Autodesk Fusion 360 part; units mm, degrees
(part 2 of 2)
  spline S17 degree 5 poles (28.5555, 1.0566) (28.5421, 1.0647) (28.5154, 1.0808) (28.4753, 1.1049) (28.4218, 1.1368) (28.3548, 1.1763) (28.2877, 1.2154) (28.2205, 1.2541) (28.1532, 1.2924) (28.0858, 1.3303) (28.0183, 1.3678) (27.9507, 1.4049) (27.883, 1.4416) (27.8153, 1.4778) (27.7474, 1.5136) (27.6795, 1.549) (27.6114, 1.584) (27.5433, 1.6186) (27.4751, 1.6527) (27.4068, 1.6864) (27.3384, 1.7197) (27.27, 1.7525) (27.2015, 1.7849) (27.1329, 1.8169) (27.0642, 1.8484) (26.9954, 1.8794) (26.9266, 1.91) (26.8577, 1.9401) (26.7887, 1.9698) (26.7197, 1.999) (26.6506, 2.0277) (26.5814, 2.056) (26.5122, 2.0837) (26.4429, 2.111) (26.3735, 2.1378) (26.3041, 2.1641) (26.2347, 2.1899) (26.1651, 2.2152) (26.0955, 2.24) (26.0259, 2.2643) (25.9562, 2.288) (25.8865, 2.3112) (25.8167, 2.3339) (25.7469, 2.356) (25.677, 2.3776) (25.6071, 2.3986) (25.5372, 2.4191) (25.4672, 2.4389) (25.3972, 2.4583) (25.3272, 2.477) (25.2571, 2.4951) (25.187, 2.5126) (25.1169, 2.5294) (25.0467, 2.5455) (24.9766, 2.5609) (24.9064, 2.5757) (24.8362, 2.5899) (24.766, 2.6035) (24.6958, 2.6165) (24.6256, 2.6287) (24.5554, 2.6401) (24.4852, 2.6504) (24.415, 2.6597) (24.3448, 2.6678) (24.2747, 2.6751) (24.2046, 2.6816) (24.1345, 2.6875) (24.0645, 2.693) (23.9945, 2.6977) (23.9245, 2.701) (23.8548, 2.7021) (23.7991, 2.7005) (23.7574, 2.6976) (23.7296, 2.6948) (23.7158, 2.6932) knots -1 -1 -1 -1 -1 -1 -0.98571429 -0.97142857 -0.95714286 -0.94285714 -0.92857143 -0.91428571 -0.9 -0.88571429 -0.87142857 -0.85714286 -0.84285714 -0.82857143 -0.81428571 -0.8 -0.78571429 -0.77142857 -0.75714286 -0.74285714 -0.72857143 -0.71428571 -0.7 -0.68571429 -0.67142857 -0.65714286 -0.64285714 -0.62857143 -0.61428571 -0.6 -0.58571429 -0.57142857 -0.55714286 -0.54285714 -0.52857143 -0.51428571 -0.5 -0.48571429 -0.47142857 -0.45714286 -0.44285714 -0.42857143 -0.41428571 -0.4 -0.38571429 -0.37142857 -0.35714286 -0.34285714 -0.32857143 -0.31428571 -0.3 -0.28571429 -0.27142857 -0.25714286 -0.24285714 -0.22857143 -0.21428571 -0.2 -0.18571429 -0.17142857 -0.15714286 -0.14285714 -0.12857143 -0.11428571 -0.1 -0.08571429 -0.07142857 -0.05714286 -0.04285714 -0.02857143 -0.01428571 0 0 0 0 0 0
  line L17 (23.7158, 2.6932) -> (22.924, 2.6037)
  arc A35 (21.1843, 3.8942) -> (22.924, 2.6037) centre (22.7456, 4.1812) ccw
  arc A36 (21.1843, 3.8942) -> (21.0619, 4.5091) centre (0, 0) ccw
  arc A37 (22.1754, 6.3671) -> (21.0619, 4.5091) centre (22.6143, 4.8415) ccw
  line L18 (22.1754, 6.3671) -> (22.9412, 6.5874)
  spline S18 degree 5 poles (22.9412, 6.5874) (22.9546, 6.5912) (22.9813, 6.5993) (23.0209, 6.6126) (23.073, 6.6324) (23.137, 6.6601) (23.2003, 6.69) (23.2632, 6.7211) (23.3258, 6.7529) (23.3883, 6.7853) (23.4506, 6.8181) (23.5126, 6.8516) (23.5743, 6.886) (23.6356, 6.9214) (23.6965, 6.9578) (23.757, 6.9952) (23.8172, 7.0334) (23.8771, 7.0722) (23.9368, 7.1116) (23.9962, 7.1516) (24.0554, 7.1921) (24.1143, 7.2332) (24.1729, 7.2749) (24.2313, 7.3173) (24.2893, 7.3603) (24.3472, 7.4038) (24.4047, 7.4479) (24.462, 7.4926) (24.519, 7.5377) (24.5758, 7.5834) (24.6323, 7.6296) (24.6886, 7.6762) (24.7447, 7.7234) (24.8005, 7.771) (24.856, 7.8192) (24.9113, 7.8678) (24.9663, 7.9168) (25.0211, 7.9664) (25.0757, 8.0163) (25.13, 8.0668) (25.1841, 8.1176) (25.2379, 8.1689) (25.2915, 8.2206) (25.3448, 8.2728) (25.3979, 8.3254) (25.4508, 8.3784) (25.5034, 8.4318) (25.5557, 8.4856) (25.6079, 8.5398) (25.6597, 8.5944) (25.7114, 8.6493) (25.7628, 8.7047) (25.8139, 8.7605) (25.8649, 8.8166) (25.9155, 8.8732) (25.966, 8.9301) (26.0162, 8.9873) (26.0661, 9.045) (26.1158, 9.103) (26.1653, 9.1613) (26.2145, 9.2201) (26.2635, 9.2791) (26.3122, 9.3386) (26.3607, 9.3983) (26.409, 9.4584) (26.457, 9.5189) (26.5047, 9.5797) (26.5523, 9.6408) (26.5995, 9.7023) (26.6466, 9.7641) (26.6933, 9.8262) (26.7306, 9.8762) (26.7584, 9.9138) (26.7769, 9.939) (26.7861, 9.9516) knots 0 0 0 0 0 0 0.01428571 0.02857143 0.04285714 0.05714286 0.07142857 0.08571429 0.1 0.11428571 0.12857143 0.14285714 0.15714286 0.17142857 0.18571429 0.2 0.21428571 0.22857143 0.24285714 0.25714286 0.27142857 0.28571429 0.3 0.31428571 0.32857143 0.34285714 0.35714286 0.37142857 0.38571429 0.4 0.41428571 0.42857143 0.44285714 0.45714286 0.47142857 0.48571429 0.5 0.51428571 0.52857143 0.54285714 0.55714286 0.57142857 0.58571429 0.6 0.61428571 0.62857143 0.64285714 0.65714286 0.67142857 0.68571429 0.7 0.71428571 0.72857143 0.74285714 0.75714286 0.77142857 0.78571429 0.8 0.81428571 0.82857143 0.84285714 0.85714286 0.87142857 0.88571429 0.9 0.91428571 0.92857143 0.94285714 0.95714286 0.97142857 0.98571429 1 1 1 1 1 1
  arc A38 (26.7861, 9.9516) -> (25.9775, 11.9038) centre (0, 0) ccw
  spline S19 degree 5 poles (25.9775, 11.9038) (25.962, 11.9062) (25.9312, 11.9109) (25.8849, 11.9178) (25.8232, 11.9268) (25.7462, 11.9377) (25.6693, 11.9481) (25.5924, 11.9582) (25.5156, 11.9678) (25.4388, 11.977) (25.3621, 11.9858) (25.2855, 11.9942) (25.2089, 12.0022) (25.1324, 12.0098) (25.056, 12.0169) (24.9797, 12.0236) (24.9034, 12.0299) (24.8273, 12.0358) (24.7512, 12.0412) (24.6752, 12.0462) (24.5993, 12.0508) (24.5235, 12.0549) (24.4478, 12.0586) (24.3722, 12.0619) (24.2967, 12.0647) (24.2213, 12.0671) (24.146, 12.069) (24.0708, 12.0704) (23.9958, 12.0715) (23.9208, 12.072) (23.846, 12.0721) (23.7712, 12.0717) (23.6967, 12.0709) (23.6222, 12.0696) (23.5479, 12.0678) (23.4737, 12.0655) (23.3996, 12.0628) (23.3257, 12.0595) (23.2519, 12.0558) (23.1783, 12.0516) (23.1048, 12.0469) (23.0315, 12.0416) (22.9584, 12.0359) (22.8854, 12.0296) (22.8126, 12.0228) (22.74, 12.0154) (22.6676, 12.0076) (22.5953, 11.9992) (22.5232, 11.9902) (22.4513, 11.9808) (22.3796, 11.9707) (22.3082, 11.96) (22.237, 11.9487) (22.166, 11.9367) (22.0953, 11.9241) (22.0248, 11.9109) (21.9545, 11.8972) (21.8845, 11.8829) (21.8146, 11.868) (21.7451, 11.8524) (21.6759, 11.836) (21.6071, 11.8187) (21.5387, 11.8004) (21.4708, 11.7811) (21.4032, 11.761) (21.3359, 11.7401) (21.2689, 11.7188) (21.2021, 11.697) (21.1356, 11.6746) (21.0698, 11.6509) (21.0049, 11.6252) (20.954, 11.6024) (20.9166, 11.5838) (20.8921, 11.5706) (20.8798, 11.5639) knots -1 -1 -1 -1 -1 -1 -0.98571429 -0.97142857 -0.95714286 -0.94285714 -0.92857143 -0.91428571 -0.9 -0.88571429 -0.87142857 -0.85714286 -0.84285714 -0.82857143 -0.81428571 -0.8 -0.78571429 -0.77142857 -0.75714286 -0.74285714 -0.72857143 -0.71428571 -0.7 -0.68571429 -0.67142857 -0.65714286 -0.64285714 -0.62857143 -0.61428571 -0.6 -0.58571429 -0.57142857 -0.55714286 -0.54285714 -0.52857143 -0.51428571 -0.5 -0.48571429 -0.47142857 -0.45714286 -0.44285714 -0.42857143 -0.41428571 -0.4 -0.38571429 -0.37142857 -0.35714286 -0.34285714 -0.32857143 -0.31428571 -0.3 -0.28571429 -0.27142857 -0.25714286 -0.24285714 -0.22857143 -0.21428571 -0.2 -0.18571429 -0.17142857 -0.15714286 -0.14285714 -0.12857143 -0.11428571 -0.1 -0.08571429 -0.07142857 -0.05714286 -0.04285714 -0.02857143 -0.01428571 0 0 0 0 0 0
  line L19 (20.8798, 11.5639) -> (20.1826, 11.1781)
  arc A39 (18.0815, 11.7046) -> (20.1826, 11.1781) centre (19.4141, 12.5673) ccw
  arc A40 (18.0815, 11.7046) -> (17.7331, 12.226) centre (0, 0) ccw
  arc A41 (18.0508, 14.3686) -> (17.7331, 12.226) centre (19.0401, 13.127) ccw
  line L20 (18.0508, 14.3686) -> (18.674, 14.8652)
  spline S20 degree 5 poles (18.674, 14.8652) (18.6849, 14.8739) (18.7065, 14.8915) (18.738, 14.919) (18.7785, 14.9572) (18.8271, 15.0073) (18.8742, 15.0591) (18.9204, 15.1119) (18.966, 15.1653) (19.0114, 15.2191) (19.0564, 15.2733) (19.1008, 15.3279) (19.1447, 15.3833) (19.1877, 15.4395) (19.2301, 15.4965) (19.2717, 15.5541) (19.3127, 15.6124) (19.3532, 15.6712) (19.3932, 15.7305) (19.4328, 15.7902) (19.472, 15.8502) (19.5106, 15.9108) (19.5489, 15.9717) (19.5866, 16.0332) (19.6238, 16.0951) (19.6605, 16.1575) (19.6968, 16.2203) (19.7326, 16.2834) (19.768, 16.347) (19.803, 16.4109) (19.8376, 16.4752) (19.8718, 16.5398) (19.9055, 16.6049) (19.9388, 16.6702) (19.9717, 16.7359) (20.0042, 16.802) (20.0363, 16.8684) (20.0679, 16.9351) (20.0992, 17.0022) (20.1301, 17.0696) (20.1606, 17.1372) (20.1907, 17.2052) (20.2204, 17.2735) (20.2497, 17.3421) (20.2786, 17.411) (20.3072, 17.4802) (20.3354, 17.5496) (20.3631, 17.6194) (20.3906, 17.6894) (20.4176, 17.7597) (20.4443, 17.8303) (20.4706, 17.9011) (20.4965, 17.9722) (20.522, 18.0436) (20.5472, 18.1152) (20.572, 18.1871) (20.5965, 18.2592) (20.6206, 18.3315) (20.6443, 18.4041) (20.6677, 18.477) (20.6907, 18.5501) (20.7133, 18.6234) (20.7356, 18.6969) (20.7575, 18.7707) (20.7791, 18.8447) (20.8003, 18.919) (20.8212, 18.9934) (20.8417, 19.0681) (20.8618, 19.143) (20.8817, 19.2181) (20.9011, 19.2934) (20.9164, 19.3538) (20.9277, 19.3992) (20.9351, 19.4295) (20.9389, 19.4447) knots 0 0 0 0 0 0 0.01428571 0.02857143 0.04285714 0.05714286 0.07142857 0.08571429 0.1 0.11428571 0.12857143 0.14285714 0.15714286 0.17142857 0.18571429 0.2 0.21428571 0.22857143 0.24285714 0.25714286 0.27142857 0.28571429 0.3 0.31428571 0.32857143 0.34285714 0.35714286 0.37142857 0.38571429 0.4 0.41428571 0.42857143 0.44285714 0.45714286 0.47142857 0.48571429 0.5 0.51428571 0.52857143 0.54285714 0.55714286 0.57142857 0.58571429 0.6 0.61428571 0.62857143 0.64285714 0.65714286 0.67142857 0.68571429 0.7 0.71428571 0.72857143 0.74285714 0.75714286 0.77142857 0.78571429 0.8 0.81428571 0.82857143 0.84285714 0.85714286 0.87142857 0.88571429 0.9 0.91428571 0.92857143 0.94285714 0.95714286 0.97142857 0.98571429 1 1 1 1 1 1
  arc A42 (20.9389, 19.4447) -> (19.4447, 20.9389) centre (0, 0) ccw
  spline S21 degree 5 poles (19.4447, 20.9389) (19.4295, 20.9351) (19.3992, 20.9277) (19.3538, 20.9164) (19.2934, 20.9011) (19.2181, 20.8817) (19.143, 20.8618) (19.0681, 20.8417) (18.9934, 20.8212) (18.919, 20.8003) (18.8447, 20.7791) (18.7707, 20.7575) (18.6969, 20.7356) (18.6234, 20.7133) (18.5501, 20.6907) (18.477, 20.6677) (18.4041, 20.6443) (18.3315, 20.6206) (18.2592, 20.5965) (18.1871, 20.572) (18.1152, 20.5472) (18.0436, 20.522) (17.9722, 20.4965) (17.9011, 20.4706) (17.8303, 20.4443) (17.7597, 20.4176) (17.6894, 20.3906) (17.6194, 20.3631) (17.5496, 20.3354) (17.4802, 20.3072) (17.411, 20.2786) (17.3421, 20.2497) (17.2735, 20.2204) (17.2052, 20.1907) (17.1372, 20.1606) (17.0696, 20.1301) (17.0022, 20.0992) (16.9351, 20.0679) (16.8684, 20.0363) (16.802, 20.0042) (16.7359, 19.9717) (16.6702, 19.9388) (16.6049, 19.9055) (16.5398, 19.8718) (16.4752, 19.8376) (16.4109, 19.803) (16.347, 19.768) (16.2834, 19.7326) (16.2203, 19.6968) (16.1575, 19.6605) (16.0951, 19.6238) (16.0332, 19.5866) (15.9717, 19.5489) (15.9108, 19.5106) (15.8502, 19.472) (15.7902, 19.4328) (15.7305, 19.3932) (15.6712, 19.3532) (15.6124, 19.3127) (15.5541, 19.2717) (15.4965, 19.2301) (15.4395, 19.1877) (15.3833, 19.1447) (15.3279, 19.1008) (15.2733, 19.0564) (15.2191, 19.0114) (15.1653, 18.966) (15.1119, 18.9204) (15.0591, 18.8742) (15.0073, 18.8271) (14.9572, 18.7785) (14.919, 18.738) (14.8915, 18.7065) (14.8739, 18.6849) (14.8652, 18.674) knots -1 -1 -1 -1 -1 -1 -0.98571429 -0.97142857 -0.95714286 -0.94285714 -0.92857143 -0.91428571 -0.9 -0.88571429 -0.87142857 -0.85714286 -0.84285714 -0.82857143 -0.81428571 -0.8 -0.78571429 -0.77142857 -0.75714286 -0.74285714 -0.72857143 -0.71428571 -0.7 -0.68571429 -0.67142857 -0.65714286 -0.64285714 -0.62857143 -0.61428571 -0.6 -0.58571429 -0.57142857 -0.55714286 -0.54285714 -0.52857143 -0.51428571 -0.5 -0.48571429 -0.47142857 -0.45714286 -0.44285714 -0.42857143 -0.41428571 -0.4 -0.38571429 -0.37142857 -0.35714286 -0.34285714 -0.32857143 -0.31428571 -0.3 -0.28571429 -0.27142857 -0.25714286 -0.24285714 -0.22857143 -0.21428571 -0.2 -0.18571429 -0.17142857 -0.15714286 -0.14285714 -0.12857143 -0.11428571 -0.1 -0.08571429 -0.07142857 -0.05714286 -0.04285714 -0.02857143 -0.01428571 0 0 0 0 0 0
  line L21 (14.8652, 18.674) -> (14.3686, 18.0508)
  arc A43 (12.226, 17.7331) -> (14.3686, 18.0508) centre (13.127, 19.0401) ccw
  arc A44 (12.226, 17.7331) -> (11.7046, 18.0815) centre (0, 0) ccw
  arc A45 (11.1781, 20.1826) -> (11.7046, 18.0815) centre (12.5673, 19.4141) ccw
  line L22 (11.1781, 20.1826) -> (11.5639, 20.8798)
  spline S22 degree 5 poles (11.5639, 20.8798) (11.5706, 20.8921) (11.5838, 20.9166) (11.6024, 20.954) (11.6252, 21.0049) (11.6509, 21.0698) (11.6746, 21.1356) (11.697, 21.2021) (11.7188, 21.2689) (11.7401, 21.3359) (11.761, 21.4032) (11.7811, 21.4708) (11.8004, 21.5387) (11.8187, 21.6071) (11.836, 21.6759) (11.8524, 21.7451) (11.868, 21.8146) (11.8829, 21.8845) (11.8972, 21.9545) (11.9109, 22.0248) (11.9241, 22.0953) (11.9367, 22.166) (11.9487, 22.237) (11.96, 22.3082) (11.9707, 22.3796) (11.9808, 22.4513) (11.9902, 22.5232) (11.9992, 22.5953) (12.0076, 22.6676) (12.0154, 22.74) (12.0228, 22.8126) (12.0296, 22.8854) (12.0359, 22.9584) (12.0416, 23.0315) (12.0469, 23.1048) (12.0516, 23.1783) (12.0558, 23.2519) (12.0595, 23.3257) (12.0628, 23.3996) (12.0655, 23.4737) (12.0678, 23.5479) (12.0696, 23.6222) (12.0709, 23.6967) (12.0717, 23.7712) (12.0721, 23.846) (12.072, 23.9208) (12.0715, 23.9958) (12.0704, 24.0708) (12.069, 24.146) (12.0671, 24.2213) (12.0647, 24.2967) (12.0619, 24.3722) (12.0586, 24.4478) (12.0549, 24.5235) (12.0508, 24.5993) (12.0462, 24.6752) (12.0412, 24.7512) (12.0358, 24.8273) (12.0299, 24.9034) (12.0236, 24.9797) (12.0169, 25.056) (12.0098, 25.1324) (12.0022, 25.2089) (11.9942, 25.2855) (11.9858, 25.3621) (11.977, 25.4388) (11.9678, 25.5156) (11.9582, 25.5924) (11.9481, 25.6693) (11.9377, 25.7462) (11.9268, 25.8232) (11.9178, 25.8849) (11.9109, 25.9312) (11.9062, 25.962) (11.9038, 25.9775) knots 0 0 0 0 0 0 0.01428571 0.02857143 0.04285714 0.05714286 0.07142857 0.08571429 0.1 0.11428571 0.12857143 0.14285714 0.15714286 0.17142857 0.18571429 0.2 0.21428571 0.22857143 0.24285714 0.25714286 0.27142857 0.28571429 0.3 0.31428571 0.32857143 0.34285714 0.35714286 0.37142857 0.38571429 0.4 0.41428571 0.42857143 0.44285714 0.45714286 0.47142857 0.48571429 0.5 0.51428571 0.52857143 0.54285714 0.55714286 0.57142857 0.58571429 0.6 0.61428571 0.62857143 0.64285714 0.65714286 0.67142857 0.68571429 0.7 0.71428571 0.72857143 0.74285714 0.75714286 0.77142857 0.78571429 0.8 0.81428571 0.82857143 0.84285714 0.85714286 0.87142857 0.88571429 0.9 0.91428571 0.92857143 0.94285714 0.95714286 0.97142857 0.98571429 1 1 1 1 1 1
  arc A46 (11.9038, 25.9775) -> (9.9516, 26.7861) centre (0, 0) ccw
  spline S23 degree 5 poles (9.9516, 26.7861) (9.939, 26.7769) (9.9138, 26.7584) (9.8762, 26.7306) (9.8262, 26.6933) (9.7641, 26.6466) (9.7023, 26.5995) (9.6408, 26.5523) (9.5797, 26.5047) (9.5189, 26.457) (9.4584, 26.409) (9.3983, 26.3607) (9.3386, 26.3122) (9.2791, 26.2635) (9.2201, 26.2145) (9.1613, 26.1653) (9.103, 26.1158) (9.045, 26.0661) (8.9873, 26.0162) (8.9301, 25.966) (8.8732, 25.9155) (8.8166, 25.8649) (8.7605, 25.8139) (8.7047, 25.7628) (8.6493, 25.7114) (8.5944, 25.6597) (8.5398, 25.6079) (8.4856, 25.5557) (8.4318, 25.5034) (8.3784, 25.4508) (8.3254, 25.3979) (8.2728, 25.3448) (8.2206, 25.2915) (8.1689, 25.2379) (8.1176, 25.1841) (8.0668, 25.13) (8.0163, 25.0757) (7.9664, 25.0211) (7.9168, 24.9663) (7.8678, 24.9113) (7.8192, 24.856) (7.771, 24.8005) (7.7234, 24.7447) (7.6762, 24.6886) (7.6296, 24.6323) (7.5834, 24.5758) (7.5377, 24.519) (7.4926, 24.462) (7.4479, 24.4047) (7.4038, 24.3472) (7.3603, 24.2893) (7.3173, 24.2313) (7.2749, 24.1729) (7.2332, 24.1143) (7.1921, 24.0554) (7.1516, 23.9962) (7.1116, 23.9368) (7.0722, 23.8771) (7.0334, 23.8172) (6.9952, 23.757) (6.9578, 23.6965) (6.9214, 23.6356) (6.886, 23.5743) (6.8516, 23.5126) (6.8181, 23.4506) (6.7853, 23.3883) (6.7529, 23.3258) (6.7211, 23.2632) (6.69, 23.2003) (6.6601, 23.137) (6.6324, 23.073) (6.6126, 23.0209) (6.5993, 22.9813) (6.5912, 22.9546) (6.5874, 22.9412) knots -1 -1 -1 -1 -1 -1 -0.98571429 -0.97142857 -0.95714286 -0.94285714 -0.92857143 -0.91428571 -0.9 -0.88571429 -0.87142857 -0.85714286 -0.84285714 -0.82857143 -0.81428571 -0.8 -0.78571429 -0.77142857 -0.75714286 -0.74285714 -0.72857143 -0.71428571 -0.7 -0.68571429 -0.67142857 -0.65714286 -0.64285714 -0.62857143 -0.61428571 -0.6 -0.58571429 -0.57142857 -0.55714286 -0.54285714 -0.52857143 -0.51428571 -0.5 -0.48571429 -0.47142857 -0.45714286 -0.44285714 -0.42857143 -0.41428571 -0.4 -0.38571429 -0.37142857 -0.35714286 -0.34285714 -0.32857143 -0.31428571 -0.3 -0.28571429 -0.27142857 -0.25714286 -0.24285714 -0.22857143 -0.21428571 -0.2 -0.18571429 -0.17142857 -0.15714286 -0.14285714 -0.12857143 -0.11428571 -0.1 -0.08571429 -0.07142857 -0.05714286 -0.04285714 -0.02857143 -0.01428571 0 0 0 0 0 0
  line L23 (6.5874, 22.9412) -> (6.3671, 22.1754)
  arc A47 (4.5091, 21.0619) -> (6.3671, 22.1754) centre (4.8415, 22.6143) ccw
  arc A48 (4.5091, 21.0619) -> (3.8942, 21.1843) centre (0, 0) ccw
  arc A49 (2.6037, 22.924) -> (3.8942, 21.1843) centre (4.1812, 22.7456) ccw
  line L24 (2.6037, 22.924) -> (2.6932, 23.7158)
  spline S24 degree 5 poles (2.6932, 23.7158) (2.6948, 23.7296) (2.6976, 23.7574) (2.7005, 23.7991) (2.7021, 23.8548) (2.701, 23.9245) (2.6977, 23.9945) (2.693, 24.0645) (2.6875, 24.1345) (2.6816, 24.2046) (2.6751, 24.2747) (2.6678, 24.3448) (2.6597, 24.415) (2.6504, 24.4852) (2.6401, 24.5554) (2.6287, 24.6256) (2.6165, 24.6958) (2.6035, 24.766) (2.5899, 24.8362) (2.5757, 24.9064) (2.5609, 24.9766) (2.5455, 25.0467) (2.5294, 25.1169) (2.5126, 25.187) (2.4951, 25.2571) (2.477, 25.3272) (2.4583, 25.3972) (2.4389, 25.4672) (2.4191, 25.5372) (2.3986, 25.6071) (2.3776, 25.677) (2.356, 25.7469) (2.3339, 25.8167) (2.3112, 25.8865) (2.288, 25.9562) (2.2643, 26.0259) (2.24, 26.0955) (2.2152, 26.1651) (2.1899, 26.2347) (2.1641, 26.3041) (2.1378, 26.3735) (2.111, 26.4429) (2.0837, 26.5122) (2.056, 26.5814) (2.0277, 26.6506) (1.999, 26.7197) (1.9698, 26.7887) (1.9401, 26.8577) (1.91, 26.9266) (1.8794, 26.9954) (1.8484, 27.0642) (1.8169, 27.1329) (1.7849, 27.2015) (1.7525, 27.27) (1.7197, 27.3384) (1.6864, 27.4068) (1.6527, 27.4751) (1.6186, 27.5433) (1.584, 27.6114) (1.549, 27.6795) (1.5136, 27.7474) (1.4778, 27.8153) (1.4416, 27.883) (1.4049, 27.9507) (1.3678, 28.0183) (1.3303, 28.0858) (1.2924, 28.1532) (1.2541, 28.2205) (1.2154, 28.2877) (1.1763, 28.3548) (1.1368, 28.4218) (1.1049, 28.4753) (1.0808, 28.5154) (1.0647, 28.5421) (1.0566, 28.5555) knots 0 0 0 0 0 0 0.01428571 0.02857143 0.04285714 0.05714286 0.07142857 0.08571429 0.1 0.11428571 0.12857143 0.14285714 0.15714286 0.17142857 0.18571429 0.2 0.21428571 0.22857143 0.24285714 0.25714286 0.27142857 0.28571429 0.3 0.31428571 0.32857143 0.34285714 0.35714286 0.37142857 0.38571429 0.4 0.41428571 0.42857143 0.44285714 0.45714286 0.47142857 0.48571429 0.5 0.51428571 0.52857143 0.54285714 0.55714286 0.57142857 0.58571429 0.6 0.61428571 0.62857143 0.64285714 0.65714286 0.67142857 0.68571429 0.7 0.71428571 0.72857143 0.74285714 0.75714286 0.77142857 0.78571429 0.8 0.81428571 0.82857143 0.84285714 0.85714286 0.87142857 0.88571429 0.9 0.91428571 0.92857143 0.94285714 0.95714286 0.97142857 0.98571429 1 1 1 1 1 1
  arc A50 (1.0566, 28.5555) -> (-1.0566, 28.5555) centre (0, 0) ccw
  spline S25 degree 5 poles (-1.0566, 28.5555) (-1.0647, 28.5421) (-1.0808, 28.5154) (-1.1049, 28.4753) (-1.1368, 28.4218) (-1.1763, 28.3548) (-1.2154, 28.2877) (-1.2541, 28.2205) (-1.2924, 28.1532) (-1.3303, 28.0858) (-1.3678, 28.0183) (-1.4049, 27.9507) (-1.4416, 27.883) (-1.4778, 27.8153) (-1.5136, 27.7474) (-1.549, 27.6795) (-1.584, 27.6114) (-1.6186, 27.5433) (-1.6527, 27.4751) (-1.6864, 27.4068) (-1.7197, 27.3384) (-1.7525, 27.27) (-1.7849, 27.2015) (-1.8169, 27.1329) (-1.8484, 27.0642) (-1.8794, 26.9954) (-1.91, 26.9266) (-1.9401, 26.8577) (-1.9698, 26.7887) (-1.999, 26.7197) (-2.0277, 26.6506) (-2.056, 26.5814) (-2.0837, 26.5122) (-2.111, 26.4429) (-2.1378, 26.3735) (-2.1641, 26.3041) (-2.1899, 26.2347) (-2.2152, 26.1651) (-2.24, 26.0955) (-2.2643, 26.0259) (-2.288, 25.9562) (-2.3112, 25.8865) (-2.3339, 25.8167) (-2.356, 25.7469) (-2.3776, 25.677) (-2.3986, 25.6071) (-2.4191, 25.5372) (-2.4389, 25.4672) (-2.4583, 25.3972) (-2.477, 25.3272) (-2.4951, 25.2571) (-2.5126, 25.187) (-2.5294, 25.1169) (-2.5455, 25.0467) (-2.5609, 24.9766) (-2.5757, 24.9064) (-2.5899, 24.8362) (-2.6035, 24.766) (-2.6165, 24.6958) (-2.6287, 24.6256) (-2.6401, 24.5554) (-2.6504, 24.4852) (-2.6597, 24.415) (-2.6678, 24.3448) (-2.6751, 24.2747) (-2.6816, 24.2046) (-2.6875, 24.1345) (-2.693, 24.0645) (-2.6977, 23.9945) (-2.701, 23.9245) (-2.7021, 23.8548) (-2.7005, 23.7991) (-2.6976, 23.7574) (-2.6948, 23.7296) (-2.6932, 23.7158) knots -1 -1 -1 -1 -1 -1 -0.98571429 -0.97142857 -0.95714286 -0.94285714 -0.92857143 -0.91428571 -0.9 -0.88571429 -0.87142857 -0.85714286 -0.84285714 -0.82857143 -0.81428571 -0.8 -0.78571429 -0.77142857 -0.75714286 -0.74285714 -0.72857143 -0.71428571 -0.7 -0.68571429 -0.67142857 -0.65714286 -0.64285714 -0.62857143 -0.61428571 -0.6 -0.58571429 -0.57142857 -0.55714286 -0.54285714 -0.52857143 -0.51428571 -0.5 -0.48571429 -0.47142857 -0.45714286 -0.44285714 -0.42857143 -0.41428571 -0.4 -0.38571429 -0.37142857 -0.35714286 -0.34285714 -0.32857143 -0.31428571 -0.3 -0.28571429 -0.27142857 -0.25714286 -0.24285714 -0.22857143 -0.21428571 -0.2 -0.18571429 -0.17142857 -0.15714286 -0.14285714 -0.12857143 -0.11428571 -0.1 -0.08571429 -0.07142857 -0.05714286 -0.04285714 -0.02857143 -0.01428571 0 0 0 0 0 0
  line L25 (-2.6932, 23.7158) -> (-2.6037, 22.924)
  arc A51 (-3.8942, 21.1843) -> (-2.6037, 22.924) centre (-4.1812, 22.7456) ccw
  arc A52 (-3.8942, 21.1843) -> (-4.5091, 21.0619) centre (0, 0) ccw
  arc A53 (-6.3671, 22.1754) -> (-4.5091, 21.0619) centre (-4.8415, 22.6143) ccw
  line L26 (-6.3671, 22.1754) -> (-6.5874, 22.9412)
  spline S26 degree 5 poles (-6.5874, 22.9412) (-6.5912, 22.9546) (-6.5993, 22.9813) (-6.6126, 23.0209) (-6.6324, 23.073) (-6.6601, 23.137) (-6.69, 23.2003) (-6.7211, 23.2632) (-6.7529, 23.3258) (-6.7853, 23.3883) (-6.8181, 23.4506) (-6.8516, 23.5126) (-6.886, 23.5743) (-6.9214, 23.6356) (-6.9578, 23.6965) (-6.9952, 23.757) (-7.0334, 23.8172) (-7.0722, 23.8771) (-7.1116, 23.9368) (-7.1516, 23.9962) (-7.1921, 24.0554) (-7.2332, 24.1143) (-7.2749, 24.1729) (-7.3173, 24.2313) (-7.3603, 24.2893) (-7.4038, 24.3472) (-7.4479, 24.4047) (-7.4926, 24.462) (-7.5377, 24.519) (-7.5834, 24.5758) (-7.6296, 24.6323) (-7.6762, 24.6886) (-7.7234, 24.7447) (-7.771, 24.8005) (-7.8192, 24.856) (-7.8678, 24.9113) (-7.9168, 24.9663) (-7.9664, 25.0211) (-8.0163, 25.0757) (-8.0668, 25.13) (-8.1176, 25.1841) (-8.1689, 25.2379) (-8.2206, 25.2915) (-8.2728, 25.3448) (-8.3254, 25.3979) (-8.3784, 25.4508) (-8.4318, 25.5034) (-8.4856, 25.5557) (-8.5398, 25.6079) (-8.5944, 25.6597) (-8.6493, 25.7114) (-8.7047, 25.7628) (-8.7605, 25.8139) (-8.8166, 25.8649) (-8.8732, 25.9155) (-8.9301, 25.966) (-8.9873, 26.0162) (-9.045, 26.0661) (-9.103, 26.1158) (-9.1613, 26.1653) (-9.2201, 26.2145) (-9.2791, 26.2635) (-9.3386, 26.3122) (-9.3983, 26.3607) (-9.4584, 26.409) (-9.5189, 26.457) (-9.5797, 26.5047) (-9.6408, 26.5523) (-9.7023, 26.5995) (-9.7641, 26.6466) (-9.8262, 26.6933) (-9.8762, 26.7306) (-9.9138, 26.7584) (-9.939, 26.7769) (-9.9516, 26.7861) knots 0 0 0 0 0 0 0.01428571 0.02857143 0.04285714 0.05714286 0.07142857 0.08571429 0.1 0.11428571 0.12857143 0.14285714 0.15714286 0.17142857 0.18571429 0.2 0.21428571 0.22857143 0.24285714 0.25714286 0.27142857 0.28571429 0.3 0.31428571 0.32857143 0.34285714 0.35714286 0.37142857 0.38571429 0.4 0.41428571 0.42857143 0.44285714 0.45714286 0.47142857 0.48571429 0.5 0.51428571 0.52857143 0.54285714 0.55714286 0.57142857 0.58571429 0.6 0.61428571 0.62857143 0.64285714 0.65714286 0.67142857 0.68571429 0.7 0.71428571 0.72857143 0.74285714 0.75714286 0.77142857 0.78571429 0.8 0.81428571 0.82857143 0.84285714 0.85714286 0.87142857 0.88571429 0.9 0.91428571 0.92857143 0.94285714 0.95714286 0.97142857 0.98571429 1 1 1 1 1 1
  arc A54 (-9.9516, 26.7861) -> (-11.9038, 25.9775) centre (0, 0) ccw
  spline S27 degree 5 poles (-11.9038, 25.9775) (-11.9062, 25.962) (-11.9109, 25.9312) (-11.9178, 25.8849) (-11.9268, 25.8232) (-11.9377, 25.7462) (-11.9481, 25.6693) (-11.9582, 25.5924) (-11.9678, 25.5156) (-11.977, 25.4388) (-11.9858, 25.3621) (-11.9942, 25.2855) (-12.0022, 25.2089) (-12.0098, 25.1324) (-12.0169, 25.056) (-12.0236, 24.9797) (-12.0299, 24.9034) (-12.0358, 24.8273) (-12.0412, 24.7512) (-12.0462, 24.6752) (-12.0508, 24.5993) (-12.0549, 24.5235) (-12.0586, 24.4478) (-12.0619, 24.3722) (-12.0647, 24.2967) (-12.0671, 24.2213) (-12.069, 24.146) (-12.0704, 24.0708) (-12.0715, 23.9958) (-12.072, 23.9208) (-12.0721, 23.846) (-12.0717, 23.7712) (-12.0709, 23.6967) (-12.0696, 23.6222) (-12.0678, 23.5479) (-12.0655, 23.4737) (-12.0628, 23.3996) (-12.0595, 23.3257) (-12.0558, 23.2519) (-12.0516, 23.1783) (-12.0469, 23.1048) (-12.0416, 23.0315) (-12.0359, 22.9584) (-12.0296, 22.8854) (-12.0228, 22.8126) (-12.0154, 22.74) (-12.0076, 22.6676) (-11.9992, 22.5953) (-11.9902, 22.5232) (-11.9808, 22.4513) (-11.9707, 22.3796) (-11.96, 22.3082) (-11.9487, 22.237) (-11.9367, 22.166) (-11.9241, 22.0953) (-11.9109, 22.0248) (-11.8972, 21.9545) (-11.8829, 21.8845) (-11.868, 21.8146) (-11.8524, 21.7451) (-11.836, 21.6759) (-11.8187, 21.6071) (-11.8004, 21.5387) (-11.7811, 21.4708) (-11.761, 21.4032) (-11.7401, 21.3359) (-11.7188, 21.2689) (-11.697, 21.2021) (-11.6746, 21.1356) (-11.6509, 21.0698) (-11.6252, 21.0049) (-11.6024, 20.954) (-11.5838, 20.9166) (-11.5706, 20.8921) (-11.5639, 20.8798) knots -1 -1 -1 -1 -1 -1 -0.98571429 -0.97142857 -0.95714286 -0.94285714 -0.92857143 -0.91428571 -0.9 -0.88571429 -0.87142857 -0.85714286 -0.84285714 -0.82857143 -0.81428571 -0.8 -0.78571429 -0.77142857 -0.75714286 -0.74285714 -0.72857143 -0.71428571 -0.7 -0.68571429 -0.67142857 -0.65714286 -0.64285714 -0.62857143 -0.61428571 -0.6 -0.58571429 -0.57142857 -0.55714286 -0.54285714 -0.52857143 -0.51428571 -0.5 -0.48571429 -0.47142857 -0.45714286 -0.44285714 -0.42857143 -0.41428571 -0.4 -0.38571429 -0.37142857 -0.35714286 -0.34285714 -0.32857143 -0.31428571 -0.3 -0.28571429 -0.27142857 -0.25714286 -0.24285714 -0.22857143 -0.21428571 -0.2 -0.18571429 -0.17142857 -0.15714286 -0.14285714 -0.12857143 -0.11428571 -0.1 -0.08571429 -0.07142857 -0.05714286 -0.04285714 -0.02857143 -0.01428571 0 0 0 0 0 0
  line L27 (-11.5639, 20.8798) -> (-11.1781, 20.1826)
  arc A55 (-11.7046, 18.0815) -> (-11.1781, 20.1826) centre (-12.5673, 19.4141) ccw
  arc A56 (-11.7046, 18.0815) -> (-12.226, 17.7331) centre (0, 0) ccw
  arc A57 (-14.3686, 18.0508) -> (-12.226, 17.7331) centre (-13.127, 19.0401) ccw
  line L28 (-14.3686, 18.0508) -> (-14.8652, 18.674)
  spline S28 degree 5 poles (-14.8652, 18.674) (-14.8739, 18.6849) (-14.8915, 18.7065) (-14.919, 18.738) (-14.9572, 18.7785) (-15.0073, 18.8271) (-15.0591, 18.8742) (-15.1119, 18.9204) (-15.1653, 18.966) (-15.2191, 19.0114) (-15.2733, 19.0564) (-15.3279, 19.1008) (-15.3833, 19.1447) (-15.4395, 19.1877) (-15.4965, 19.2301) (-15.5541, 19.2717) (-15.6124, 19.3127) (-15.6712, 19.3532) (-15.7305, 19.3932) (-15.7902, 19.4328) (-15.8502, 19.472) (-15.9108, 19.5106) (-15.9717, 19.5489) (-16.0332, 19.5866) (-16.0951, 19.6238) (-16.1575, 19.6605) (-16.2203, 19.6968) (-16.2834, 19.7326) (-16.347, 19.768) (-16.4109, 19.803) (-16.4752, 19.8376) (-16.5398, 19.8718) (-16.6049, 19.9055) (-16.6702, 19.9388) (-16.7359, 19.9717) (-16.802, 20.0042) (-16.8684, 20.0363) (-16.9351, 20.0679) (-17.0022, 20.0992) (-17.0696, 20.1301) (-17.1372, 20.1606) (-17.2052, 20.1907) (-17.2735, 20.2204) (-17.3421, 20.2497) (-17.411, 20.2786) (-17.4802, 20.3072) (-17.5496, 20.3354) (-17.6194, 20.3631) (-17.6894, 20.3906) (-17.7597, 20.4176) (-17.8303, 20.4443) (-17.9011, 20.4706) (-17.9722, 20.4965) (-18.0436, 20.522) (-18.1152, 20.5472) (-18.1871, 20.572) (-18.2592, 20.5965) (-18.3315, 20.6206) (-18.4041, 20.6443) (-18.477, 20.6677) (-18.5501, 20.6907) (-18.6234, 20.7133) (-18.6969, 20.7356) (-18.7707, 20.7575) (-18.8447, 20.7791) (-18.919, 20.8003) (-18.9934, 20.8212) (-19.0681, 20.8417) (-19.143, 20.8618) (-19.2181, 20.8817) (-19.2934, 20.9011) (-19.3538, 20.9164) (-19.3992, 20.9277) (-19.4295, 20.9351) (-19.4447, 20.9389) knots 0 0 0 0 0 0 0.01428571 0.02857143 0.04285714 0.05714286 0.07142857 0.08571429 0.1 0.11428571 0.12857143 0.14285714 0.15714286 0.17142857 0.18571429 0.2 0.21428571 0.22857143 0.24285714 0.25714286 0.27142857 0.28571429 0.3 0.31428571 0.32857143 0.34285714 0.35714286 0.37142857 0.38571429 0.4 0.41428571 0.42857143 0.44285714 0.45714286 0.47142857 0.48571429 0.5 0.51428571 0.52857143 0.54285714 0.55714286 0.57142857 0.58571429 0.6 0.61428571 0.62857143 0.64285714 0.65714286 0.67142857 0.68571429 0.7 0.71428571 0.72857143 0.74285714 0.75714286 0.77142857 0.78571429 0.8 0.81428571 0.82857143 0.84285714 0.85714286 0.87142857 0.88571429 0.9 0.91428571 0.92857143 0.94285714 0.95714286 0.97142857 0.98571429 1 1 1 1 1 1
  arc A58 (-19.4447, 20.9389) -> (-20.9389, 19.4447) centre (0, 0) ccw
  spline S29 degree 5 poles (-20.9389, 19.4447) (-20.9351, 19.4295) (-20.9277, 19.3992) (-20.9164, 19.3538) (-20.9011, 19.2934) (-20.8817, 19.2181) (-20.8618, 19.143) (-20.8417, 19.0681) (-20.8212, 18.9934) (-20.8003, 18.919) (-20.7791, 18.8447) (-20.7575, 18.7707) (-20.7356, 18.6969) (-20.7133, 18.6234) (-20.6907, 18.5501) (-20.6677, 18.477) (-20.6443, 18.4041) (-20.6206, 18.3315) (-20.5965, 18.2592) (-20.572, 18.1871) (-20.5472, 18.1152) (-20.522, 18.0436) (-20.4965, 17.9722) (-20.4706, 17.9011) (-20.4443, 17.8303) (-20.4176, 17.7597) (-20.3906, 17.6894) (-20.3631, 17.6194) (-20.3354, 17.5496) (-20.3072, 17.4802) (-20.2786, 17.411) (-20.2497, 17.3421) (-20.2204, 17.2735) (-20.1907, 17.2052) (-20.1606, 17.1372) (-20.1301, 17.0696) (-20.0992, 17.0022) (-20.0679, 16.9351) (-20.0363, 16.8684) (-20.0042, 16.802) (-19.9717, 16.7359) (-19.9388, 16.6702) (-19.9055, 16.6049) (-19.8718, 16.5398) (-19.8376, 16.4752) (-19.803, 16.4109) (-19.768, 16.347) (-19.7326, 16.2834) (-19.6968, 16.2203) (-19.6605, 16.1575) (-19.6238, 16.0951) (-19.5866, 16.0332) (-19.5489, 15.9717) (-19.5106, 15.9108) (-19.472, 15.8502) (-19.4328, 15.7902) (-19.3932, 15.7305) (-19.3532, 15.6712) (-19.3127, 15.6124) (-19.2717, 15.5541) (-19.2301, 15.4965) (-19.1877, 15.4395) (-19.1447, 15.3833) (-19.1008, 15.3279) (-19.0564, 15.2733) (-19.0114, 15.2191) (-18.966, 15.1653) (-18.9204, 15.1119) (-18.8742, 15.0591) (-18.8271, 15.0073) (-18.7785, 14.9572) (-18.738, 14.919) (-18.7065, 14.8915) (-18.6849, 14.8739) (-18.674, 14.8652) knots -1 -1 -1 -1 -1 -1 -0.98571429 -0.97142857 -0.95714286 -0.94285714 -0.92857143 -0.91428571 -0.9 -0.88571429 -0.87142857 -0.85714286 -0.84285714 -0.82857143 -0.81428571 -0.8 -0.78571429 -0.77142857 -0.75714286 -0.74285714 -0.72857143 -0.71428571 -0.7 -0.68571429 -0.67142857 -0.65714286 -0.64285714 -0.62857143 -0.61428571 -0.6 -0.58571429 -0.57142857 -0.55714286 -0.54285714 -0.52857143 -0.51428571 -0.5 -0.48571429 -0.47142857 -0.45714286 -0.44285714 -0.42857143 -0.41428571 -0.4 -0.38571429 -0.37142857 -0.35714286 -0.34285714 -0.32857143 -0.31428571 -0.3 -0.28571429 -0.27142857 -0.25714286 -0.24285714 -0.22857143 -0.21428571 -0.2 -0.18571429 -0.17142857 -0.15714286 -0.14285714 -0.12857143 -0.11428571 -0.1 -0.08571429 -0.07142857 -0.05714286 -0.04285714 -0.02857143 -0.01428571 0 0 0 0 0 0
  line L29 (-18.674, 14.8652) -> (-18.0508, 14.3686)
  arc A59 (-17.7331, 12.226) -> (-18.0508, 14.3686) centre (-19.0401, 13.127) ccw
  arc A60 (-17.7331, 12.226) -> (-18.0815, 11.7046) centre (0, 0) ccw
  arc A61 (-20.1826, 11.1781) -> (-18.0815, 11.7046) centre (-19.4141, 12.5673) ccw
  line L30 (-20.1826, 11.1781) -> (-20.8798, 11.5639)
  spline S30 degree 5 poles (-20.8798, 11.5639) (-20.8921, 11.5706) (-20.9166, 11.5838) (-20.954, 11.6024) (-21.0049, 11.6252) (-21.0698, 11.6509) (-21.1356, 11.6746) (-21.2021, 11.697) (-21.2689, 11.7188) (-21.3359, 11.7401) (-21.4032, 11.761) (-21.4708, 11.7811) (-21.5387, 11.8004) (-21.6071, 11.8187) (-21.6759, 11.836) (-21.7451, 11.8524) (-21.8146, 11.868) (-21.8845, 11.8829) (-21.9545, 11.8972) (-22.0248, 11.9109) (-22.0953, 11.9241) (-22.166, 11.9367) (-22.237, 11.9487) (-22.3082, 11.96) (-22.3796, 11.9707) (-22.4513, 11.9808) (-22.5232, 11.9902) (-22.5953, 11.9992) (-22.6676, 12.0076) (-22.74, 12.0154) (-22.8126, 12.0228) (-22.8854, 12.0296) (-22.9584, 12.0359) (-23.0315, 12.0416) (-23.1048, 12.0469) (-23.1783, 12.0516) (-23.2519, 12.0558) (-23.3257, 12.0595) (-23.3996, 12.0628) (-23.4737, 12.0655) (-23.5479, 12.0678) (-23.6222, 12.0696) (-23.6967, 12.0709) (-23.7712, 12.0717) (-23.846, 12.0721) (-23.9208, 12.072) (-23.9958, 12.0715) (-24.0708, 12.0704) (-24.146, 12.069) (-24.2213, 12.0671) (-24.2967, 12.0647) (-24.3722, 12.0619) (-24.4478, 12.0586) (-24.5235, 12.0549) (-24.5993, 12.0508) (-24.6752, 12.0462) (-24.7512, 12.0412) (-24.8273, 12.0358) (-24.9034, 12.0299) (-24.9797, 12.0236) (-25.056, 12.0169) (-25.1324, 12.0098) (-25.2089, 12.0022) (-25.2855, 11.9942) (-25.3621, 11.9858) (-25.4388, 11.977) (-25.5156, 11.9678) (-25.5924, 11.9582) (-25.6693, 11.9481) (-25.7462, 11.9377) (-25.8232, 11.9268) (-25.8849, 11.9178) (-25.9312, 11.9109) (-25.962, 11.9062) (-25.9775, 11.9038) knots 0 0 0 0 0 0 0.01428571 0.02857143 0.04285714 0.05714286 0.07142857 0.08571429 0.1 0.11428571 0.12857143 0.14285714 0.15714286 0.17142857 0.18571429 0.2 0.21428571 0.22857143 0.24285714 0.25714286 0.27142857 0.28571429 0.3 0.31428571 0.32857143 0.34285714 0.35714286 0.37142857 0.38571429 0.4 0.41428571 0.42857143 0.44285714 0.45714286 0.47142857 0.48571429 0.5 0.51428571 0.52857143 0.54285714 0.55714286 0.57142857 0.58571429 0.6 0.61428571 0.62857143 0.64285714 0.65714286 0.67142857 0.68571429 0.7 0.71428571 0.72857143 0.74285714 0.75714286 0.77142857 0.78571429 0.8 0.81428571 0.82857143 0.84285714 0.85714286 0.87142857 0.88571429 0.9 0.91428571 0.92857143 0.94285714 0.95714286 0.97142857 0.98571429 1 1 1 1 1 1
  arc A62 (-25.9775, 11.9038) -> (-26.7861, 9.9516) centre (0, 0) ccw
  spline S31 degree 5 poles (-26.7861, 9.9516) (-26.7769, 9.939) (-26.7584, 9.9138) (-26.7306, 9.8762) (-26.6933, 9.8262) (-26.6466, 9.7641) (-26.5995, 9.7023) (-26.5523, 9.6408) (-26.5047, 9.5797) (-26.457, 9.5189) (-26.409, 9.4584) (-26.3607, 9.3983) (-26.3122, 9.3386) (-26.2635, 9.2791) (-26.2145, 9.2201) (-26.1653, 9.1613) (-26.1158, 9.103) (-26.0661, 9.045) (-26.0162, 8.9873) (-25.966, 8.9301) (-25.9155, 8.8732) (-25.8649, 8.8166) (-25.8139, 8.7605) (-25.7628, 8.7047) (-25.7114, 8.6493) (-25.6597, 8.5944) (-25.6079, 8.5398) (-25.5557, 8.4856) (-25.5034, 8.4318) (-25.4508, 8.3784) (-25.3979, 8.3254) (-25.3448, 8.2728) (-25.2915, 8.2206) (-25.2379, 8.1689) (-25.1841, 8.1176) (-25.13, 8.0668) (-25.0757, 8.0163) (-25.0211, 7.9664) (-24.9663, 7.9168) (-24.9113, 7.8678) (-24.856, 7.8192) (-24.8005, 7.771) (-24.7447, 7.7234) (-24.6886, 7.6762) (-24.6323, 7.6296) (-24.5758, 7.5834) (-24.519, 7.5377) (-24.462, 7.4926) (-24.4047, 7.4479) (-24.3472, 7.4038) (-24.2893, 7.3603) (-24.2313, 7.3173) (-24.1729, 7.2749) (-24.1143, 7.2332) (-24.0554, 7.1921) (-23.9962, 7.1516) (-23.9368, 7.1116) (-23.8771, 7.0722) (-23.8172, 7.0334) (-23.757, 6.9952) (-23.6965, 6.9578) (-23.6356, 6.9214) (-23.5743, 6.886) (-23.5126, 6.8516) (-23.4506, 6.8181) (-23.3883, 6.7853) (-23.3258, 6.7529) (-23.2632, 6.7211) (-23.2003, 6.69) (-23.137, 6.6601) (-23.073, 6.6324) (-23.0209, 6.6126) (-22.9813, 6.5993) (-22.9546, 6.5912) (-22.9412, 6.5874) knots -1 -1 -1 -1 -1 -1 -0.98571429 -0.97142857 -0.95714286 -0.94285714 -0.92857143 -0.91428571 -0.9 -0.88571429 -0.87142857 -0.85714286 -0.84285714 -0.82857143 -0.81428571 -0.8 -0.78571429 -0.77142857 -0.75714286 -0.74285714 -0.72857143 -0.71428571 -0.7 -0.68571429 -0.67142857 -0.65714286 -0.64285714 -0.62857143 -0.61428571 -0.6 -0.58571429 -0.57142857 -0.55714286 -0.54285714 -0.52857143 -0.51428571 -0.5 -0.48571429 -0.47142857 -0.45714286 -0.44285714 -0.42857143 -0.41428571 -0.4 -0.38571429 -0.37142857 -0.35714286 -0.34285714 -0.32857143 -0.31428571 -0.3 -0.28571429 -0.27142857 -0.25714286 -0.24285714 -0.22857143 -0.21428571 -0.2 -0.18571429 -0.17142857 -0.15714286 -0.14285714 -0.12857143 -0.11428571 -0.1 -0.08571429 -0.07142857 -0.05714286 -0.04285714 -0.02857143 -0.01428571 0 0 0 0 0 0
  line L31 (-22.9412, 6.5874) -> (-22.1754, 6.3671)
  arc A63 (-21.0619, 4.5091) -> (-22.1754, 6.3671) centre (-22.6143, 4.8415) ccw
  line L32 (2.3913, -1.6197) -> (-2.3712, -1.6197)
  line L33 (-2.3712, -1.6197) -> (-2.3712, 1.5991)
  line L34 (-2.3712, 1.5991) -> (2.3913, 1.5991)
  line L35 (2.3913, 1.5991) -> (2.3913, -1.6197)
  dimension "d9" = 4.7625
  constraint horizontal L32
  constraint vertical L33
  constraint horizontal L34
  constraint vertical L35
  measures "d9" distance of L32.start L32.end
extrude "Extrude3" cut sketch "Sketch1 (2)" against normal blind 19.7866 contours L32 L33 L34 L35 in component "Spur Gear (16 teeth)"
extrude "Extrude4" cut 1 faces at (0.7904, -14.6916, 9.652) along direction (0, 0, -1) blind 3.302 in component "Spur Gear (16 teeth)"
component "Spur Gear (16 teeth)" placed x (1, 0, 0) y (0, 1, 0) z (0, 0, 1) at (0, 0, 0)
